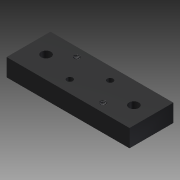
# Autodesk Inventor part: 13_0204_040
Saved by Autodesk Inventor 2014 (Build 180170000, 170)
## iProperties
Created: 2013-04-08
Part Number: 13_0204_040
Material: Allgemein
Document SubType Name: Modeling
Designer: vogel
Density: 1 g/cm^3
Appearance: Gummi - schwarz - Version 1.1
Author: vogel
Autodesk Inventor part; units mm, degrees
ref_plane "YZ Plane" through (0, 0, 0) normal (1, 0, 0) x (0, 1, 0)
ref_plane "XZ Plane" through (0, 0, 0) normal (0, 1, 0) x (-1, 0, 0)
ref_plane "XY Plane" through (0, 0, 0) normal (0, 0, 1) x (1, 0, 0)
sketch "Skizze1" plane through (0, 0, 0) normal (0, 0, 1) x (1, 0, 0)
  line L0 (-35, 12.5) -> (35, 12.5)
  line L1 (35, 12.5) -> (35, -12.5)
  line L2 (35, -12.5) -> (-35, -12.5)
  line L3 (-35, -12.5) -> (-35, 12.5)
  line L4 (-49, 0) -> (49, 0) projected
  line L5 (0, -17.5) -> (0, 17.5) projected
  point P0 (0, 0)
  dimension "d0" = 70
  dimension "d1" = 25
  constraints: 8 end point, 2 parallel, 1 horizontal, 1 perpendicular, 2 other
  measures "d0" distance of L0.start L0.end
  measures "d1" distance of L2.end L0.start
extrude "Extrusion1" add sketch "Skizze1" along normal blind 10
sketch "Skizze2" plane through (0, 0, 10) normal (0, 0, 1) x (1, 0, 0)
  line L0 (-49, 0) -> (49, 0) projected
  line L1 (0, -17.5) -> (0, 17.5) projected
  point P0 (0, 0)
  point P1 (-25, 0)
  point P2 (25, 0)
  dimension "d4" = 50
  constraints: 2 point on line, 1 symmetric about line
  measures "d4" distance of point (25, 0) point (-25, 0)
hole "Bohrung1" at (-25, 0, 10) at (25, 0, 10) direction (0, 0, -1) diameter 5 end through all
sketch "Skizze3" plane through (0, 0, 0) normal (0, 0, -1) x (-1, 0, 0)
  circle A0 centre (-25, 0) radius 2.5 projected
  circle A1 centre (25, 0) radius 2.5 projected
  point P0 (0, 0)
  constraints: 2 coincident
hole "Bohrung2" at (25, 0, 0) at (-25, 0, 0) direction (0, 0, 1) diameter 5.5 end through all counterbore diameter 10 counterbore depth 5.4
sketch "Skizze4" plane through (0, 0, 0) normal (0, 0, -1) x (-1, 0, 0)
  point P0 (6, -5.5)
hole "Bohrung3" at (-6, -5.5, 0) direction (0, 0, 1) diameter 3.4 depth 10 counterbore diameter 6.5 counterbore depth 5
sketch "Skizze5" plane through (0, 0, 0) normal (0, 0, -1) x (-1, 0, 0)
  point P0 (-6, 5.5)
hole "Bohrung5" at (6, 5.5, 0) direction (0, 0, 1) diameter 3.4 depth 10 counterbore diameter 6.5 counterbore depth 5
sketch "Skizze6" plane through (0, 0, 0) normal (0, 0, -1) x (-1, 0, 0)
  line L0 (-15, 7.5) -> (15, 7.5)
  line L1 (15, 7.5) -> (15, -7.5)
  line L2 (15, -7.5) -> (-15, -7.5)
  line L3 (-15, -7.5) -> (-15, 7.5)
  line L4 (49, 0) -> (-49, 0) projected
  line L5 (0, -17.5) -> (0, 17.5) projected
  point P0 (0, 0)
  dimension "d33" = 30
  dimension "d34" = 15
  constraints: 8 end point, 2 coincident, 2 parallel, 1 horizontal, 1 perpendicular, 2 other
  measures "d33" distance of L0.start L0.end
  measures "d34" distance of L2.end L0.start
hole "Bohrung7" at (15, -7.5, 0) at (-15, 7.5, 0) direction (0, 0, 1) diameter 3.242 end through all thread size "M4x0.7" class "6H" standard "ISO Metric profile"
